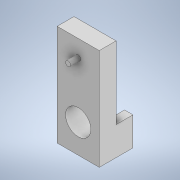
# Autodesk Inventor part: bottom_part
Saved by Autodesk Inventor 2021 (Build 250183000, 183)
## iProperties
Created: 2021-04-02
Part Number: bottom_part
Material: Generic
Document SubType Name: Modeling
Designer: Jawal
Density: 1 g/cm^3
Appearance: Default
Author: Jawal
Autodesk Inventor part; units mm, degrees
note: some values were not read from the file. Chosen so that the rebuilt part matches the saved one: direction of "Emboss1".
ref_plane "YZ Plane" through (0, 0, 0) normal (1, 0, 0) x (0, 1, 0)
ref_plane "XZ Plane" through (0, 0, 0) normal (0, 1, 0) x (-1, 0, 0)
ref_plane "XY Plane" through (0, 0, 0) normal (0, 0, 1) x (1, 0, 0)
sketch "Sketch1" plane through (0, 0, 0) normal (0, 0, 1) x (1, 0, 0)
  line L0 (-12.5, -12.5) -> (12.5, -12.5)
  line L1 (12.5, -12.5) -> (12.5, 47.5)
  line L2 (12.5, 47.5) -> (-12.5, 47.5)
  line L3 (-12.5, 47.5) -> (-12.5, -12.5)
  point P0 (0, 0)
  dimension "d0" = 60
  dimension "d1" = 25
  dimension "d2" = 12.5
  dimension "d5" = 12.5
  constraints: 8 end point, 2 parallel, 1 horizontal, 1 perpendicular
  measures "d0" distance of L0.end L1.end
  measures "d1" distance of L0.start L0.end
  measures "d2" distance from line of L3 point (0, 0)
  measures "d5" distance from line of L0 point (0, 0)
extrude "Extrusion1" add sketch "Sketch1" against normal blind 10
sketch "Sketch2" plane through (0, 0, 0) normal (0, 0, 1) x (1, 0, 0)
  circle A0 centre (0, 37.5) radius 1.5
  point P0 (0, 0)
  dimension "d8" = 3
  dimension "d29" = 37.5
  constraints: 1 centre point
  measures "d8" diameter of A0
  measures "d29" distance of point (0, 0) A0.centre
extrude "Extrusion2" add sketch "Sketch2" along normal blind 6
thread "Thread1" size "M3x0.5" class "6g" standard "ANSI Metric M Profile" full length
sketch "Sketch3" plane through (0, 0, -10) normal (0, 0, -1) x (-1, 0, 0)
  line L0 (-7.5, 4.5) -> (-12.5, 4.5)
  line L1 (-12.5, 47.5) -> (-12.5, -12.5) projected
  line L2 (-12.5, -12.5) -> (12.5, -12.5) projected
  line L3 (-12.5, -12.5) -> (12.5, -12.5)
  line L4 (12.5, -12.5) -> (12.5, 4.5)
  line L5 (12.5, -12.5) -> (12.5, 47.5) projected
  line L6 (7.5, 4.5) -> (12.5, 4.5)
  arc A0 (-7.5, 4.5) -> (7.5, 4.5) centre (0, 4.5) ccw
  point P0 (0, 0)
  dimension "d20" = 17
  dimension "d21" = 5
  dimension "d22" = 5
  dimension "d25" = 7.5
  constraints: 8 end point, 4 point on line, 2 horizontal, 2 point on circle, 1 centre point, 1 perpendicular
  measures "d20" distance of L2.end L4.end
  measures "d21" distance of L6.start L4.end
  measures "d22" distance of L0.start L0.end
  measures "d25" radius of A0
extrude "Extrusion3" add sketch "Sketch3" along normal blind 10
sketch "Sketch5" plane through (0, 0, 0) normal (0, 0, 1) x (1, 0, 0)
  circle A0 centre (0, 4.5) radius 7.5
  point P0 (0, 0)
  dimension "d26" = 15
  constraints: 1 centre point
  measures "d26" diameter of A0
extrude "Extrusion5" cut sketch "Sketch5" against normal blind 10
sketch "Sketch6" plane through (-12.5, -12.5, 0) normal (-1, 0, 0) x (0, 0, 1)
  line L0 (-17.643, 6.905) -> (1.6858, 6.905) construction
  line L1 (1.6858, 6.905) -> (1.6858, -1.4052) construction
  line L2 (1.6858, -1.4052) -> (-17.643, -1.4052) construction
  line L3 (-17.643, -1.4052) -> (-17.643, 6.905) construction
  line L4 (-17.3898, 4.3888) -> (-17.3898, 6.8888)
  line L5 (-17.3898, 6.8888) -> (-15.8257, 6.8888)
  line L6 (-15.8257, 6.8888) -> (-15.8257, 6.593)
  line L7 (-15.8257, 6.593) -> (-17.0575, 6.593)
  line L8 (-17.0575, 6.593) -> (-17.0575, 5.9082)
  line L9 (-17.0575, 5.9082) -> (-15.9088, 5.9082)
  line L10 (-15.9088, 5.9082) -> (-15.9088, 5.6124)
  line L11 (-15.9088, 5.6124) -> (-17.0575, 5.6124)
  line L12 (-17.0575, 5.6124) -> (-17.0575, 4.6846)
  line L13 (-17.0575, 4.6846) -> (-15.8257, 4.6846)
  line L14 (-15.8257, 4.6846) -> (-15.8257, 4.3888)
  line L15 (-15.8257, 4.3888) -> (-17.3898, 4.3888)
  line L16 (-14.0287, 4.3888) -> (-14.4157, 4.3888)
  line L17 (-14.4157, 4.3888) -> (-14.8715, 5.0938)
  line L18 (-14.8715, 5.0938) -> (-15.3395, 4.3888)
  line L19 (-15.3395, 4.3888) -> (-15.6981, 4.3888)
  line L20 (-15.6981, 4.3888) -> (-15.0478, 5.3187)
  line L21 (-15.0478, 5.3187) -> (-15.692, 6.2648)
  line L22 (-15.692, 6.2648) -> (-15.3051, 6.2648)
  line L23 (-15.3051, 6.2648) -> (-14.8513, 5.5658)
  line L24 (-14.8513, 5.5658) -> (-14.3873, 6.2648)
  line L25 (-14.3873, 6.2648) -> (-14.0287, 6.2648)
  line L26 (-14.0287, 6.2648) -> (-14.675, 5.3389)
  line L27 (-14.675, 5.3389) -> (-14.0287, 4.3888)
  line L28 (-13.4615, 4.3888) -> (-13.7775, 4.3888)
  line L29 (-13.7775, 4.3888) -> (-13.7775, 6.2648)
  line L30 (-13.7775, 6.2648) -> (-13.4615, 6.2648)
  line L31 (-13.4615, 6.2648) -> (-13.4615, 4.3888)
  line L32 (-13.4392, 6.5768) -> (-13.7978, 6.5768)
  line L33 (-13.7978, 6.5768) -> (-13.7978, 6.905)
  line L34 (-13.7978, 6.905) -> (-13.4392, 6.905)
  line L35 (-13.4392, 6.905) -> (-13.4392, 6.5768)
  spline S0 degree 2 poles (-12.4303, 4.3523) (-12.6876, 4.3523) (-12.9773, 4.6461) (-12.9773, 4.9641) knots 0 0 0 1 2 2 2
  line L36 (-12.9773, 4.9641) -> (-12.9773, 6.0034)
  line L37 (-12.9773, 6.0034) -> (-13.19, 6.0034)
  line L38 (-13.19, 6.0034) -> (-13.19, 6.2648)
  line L39 (-13.19, 6.2648) -> (-12.9773, 6.2648)
  line L40 (-12.9773, 6.2648) -> (-12.9773, 6.8037)
  line L41 (-12.9773, 6.8037) -> (-12.6612, 6.8037)
  line L42 (-12.6612, 6.8037) -> (-12.6612, 6.2648)
  line L43 (-12.6612, 6.2648) -> (-12.0798, 6.2648)
  line L44 (-12.0798, 6.2648) -> (-12.0798, 6.0034)
  line L45 (-12.0798, 6.0034) -> (-12.6612, 6.0034)
  line L46 (-12.6612, 6.0034) -> (-12.6612, 5.11)
  spline S1 degree 2 poles (-12.6612, 5.11) (-12.6612, 4.9682) (-12.6511, 4.8122) (-12.6167, 4.7453) knots 0 0 0 1 2 2 2
  spline S2 degree 2 poles (-12.6167, 4.7453) (-12.5883, 4.6866) (-12.4607, 4.6278) (-12.3513, 4.6278) knots 0 0 0 1 2 2 2
  spline S3 degree 2 poles (-12.3513, 4.6278) (-12.2743, 4.6278) (-12.1304, 4.6744) (-12.098, 4.6886) knots 0 0 0 1 2 2 2
  line L47 (-12.098, 4.6886) -> (-12.0798, 4.6886)
  line L48 (-12.0798, 4.6886) -> (-12.0798, 4.405)
  spline S4 degree 2 poles (-12.0798, 4.405) (-12.1689, 4.3807) (-12.3513, 4.3523) (-12.4303, 4.3523) knots 0 0 0 1 2 2 2
  line L49 (-8.814, 4.3888) -> (-9.2455, 4.3888)
  line L50 (-9.2455, 4.3888) -> (-10.0356, 5.3835)
  line L51 (-10.0356, 5.3835) -> (-10.4165, 5.3835)
  line L52 (-10.4165, 5.3835) -> (-10.4165, 4.3888)
  line L53 (-10.4165, 4.3888) -> (-10.7487, 4.3888)
  line L54 (-10.7487, 4.3888) -> (-10.7487, 6.8888)
  line L55 (-10.7487, 6.8888) -> (-10.1045, 6.8888)
  spline S5 degree 2 poles (-10.1045, 6.8888) (-9.8898, 6.8888) (-9.6, 6.8422) (-9.4684, 6.7571) knots 0 0 0 1 2 2 2
  spline S6 degree 2 poles (-9.4684, 6.7571) (-9.3367, 6.672) (-9.1847, 6.4066) (-9.1847, 6.2101) knots 0 0 0 1 2 2 2
  spline S7 degree 2 poles (-9.1847, 6.2101) (-9.1847, 5.9366) (-9.4643, 5.5658) (-9.7034, 5.4767) knots 0 0 0 1 2 2 2
  line L56 (-9.7034, 5.4767) -> (-8.814, 4.3888)
  spline S8 degree 2 poles (-9.5312, 6.1838) (-9.5312, 6.2932) (-9.6081, 6.4613) (-9.6892, 6.516) knots 0 0 0 1 2 2 2
  spline S9 degree 2 poles (-9.6892, 6.516) (-9.7601, 6.5626) (-9.9485, 6.6011) (-10.0863, 6.6011) knots 0 0 0 1 2 2 2
  line L57 (-10.0863, 6.6011) -> (-10.4165, 6.6011)
  line L58 (-10.4165, 6.6011) -> (-10.4165, 5.6611)
  line L59 (-10.4165, 5.6611) -> (-10.1248, 5.6611)
  spline S10 degree 2 poles (-10.1248, 5.6611) (-9.9809, 5.6611) (-9.752, 5.7117) (-9.673, 5.7907) knots 0 0 0 1 2 2 2
  spline S11 degree 2 poles (-9.673, 5.7907) (-9.6, 5.8596) (-9.5312, 6.0541) (-9.5312, 6.1838) knots 0 0 0 1 2 2 2
  spline S12 degree 2 poles (-7.5944, 4.5873) (-7.6329, 4.559) (-7.7625, 4.4577) (-7.8233, 4.4273) knots 0 0 0 1 2 2 2
  spline S13 degree 2 poles (-7.8233, 4.4273) (-7.9064, 4.3827) (-8.0624, 4.3361) (-8.2042, 4.3361) knots 0 0 0 1 2 2 2
  spline S14 degree 2 poles (-8.2042, 4.3361) (-8.3197, 4.3361) (-8.5283, 4.4232) (-8.6073, 4.5022) knots 0 0 0 1 2 2 2
  spline S15 degree 2 poles (-8.6073, 4.5022) (-8.6823, 4.5792) (-8.7735, 4.8061) (-8.7735, 4.9317) knots 0 0 0 1 2 2 2
  spline S16 degree 2 poles (-8.7735, 4.9317) (-8.7735, 5.1262) (-8.6094, 5.4017) (-8.4311, 5.4808) knots 0 0 0 1 2 2 2
  spline S17 degree 2 poles (-8.4311, 5.4808) (-8.2731, 5.5537) (-7.8436, 5.6084) (-7.5944, 5.6226) knots 0 0 0 1 2 2 2
  line L60 (-7.5944, 5.6226) -> (-7.5944, 5.6833)
  spline S18 degree 2 poles (-7.5944, 5.6833) (-7.5944, 5.7927) (-7.6612, 5.9285) (-7.722, 5.967) knots 0 0 0 1 2 2 2
  spline S19 degree 2 poles (-7.722, 5.967) (-7.7828, 6.0055) (-7.957, 6.0298) (-8.0502, 6.0298) knots 0 0 0 1 2 2 2
  spline S20 degree 2 poles (-8.0502, 6.0298) (-8.1596, 6.0298) (-8.4554, 5.965) (-8.6033, 5.9021) knots 0 0 0 1 2 2 2
  line L61 (-8.6033, 5.9021) -> (-8.6215, 5.9021)
  line L62 (-8.6215, 5.9021) -> (-8.6215, 6.2243)
  spline S21 degree 2 poles (-8.6215, 6.2243) (-8.5344, 6.2486) (-8.2082, 6.3094) (-8.0482, 6.3094) knots 0 0 0 1 2 2 2
  spline S22 degree 2 poles (-8.0482, 6.3094) (-7.8537, 6.3094) (-7.5883, 6.2486) (-7.4829, 6.1696) knots 0 0 0 1 2 2 2
  spline S23 degree 2 poles (-7.4829, 6.1696) (-7.3796, 6.0926) (-7.2783, 5.8474) (-7.2783, 5.6712) knots 0 0 0 1 2 2 2
  line L63 (-7.2783, 5.6712) -> (-7.2783, 4.3888)
  line L64 (-7.2783, 4.3888) -> (-7.5944, 4.3888)
  line L65 (-7.5944, 4.3888) -> (-7.5944, 4.5873)
  line L66 (-7.5944, 4.8507) -> (-7.5944, 5.3714)
  spline S24 degree 2 poles (-7.5944, 5.3714) (-7.7078, 5.3612) (-8.0502, 5.3268) (-8.1576, 5.2944) knots 0 0 0 1 2 2 2
  spline S25 degree 2 poles (-8.1576, 5.2944) (-8.2832, 5.2559) (-8.4473, 5.0958) (-8.4473, 4.954) knots 0 0 0 1 2 2 2
  spline S26 degree 2 poles (-8.4473, 4.954) (-8.4473, 4.7919) (-8.265, 4.6278) (-8.0907, 4.6278) knots 0 0 0 1 2 2 2
  spline S27 degree 2 poles (-8.0907, 4.6278) (-7.9428, 4.6278) (-7.6997, 4.7555) (-7.5944, 4.8507) knots 0 0 0 1 2 2 2
  line L67 (-4.7074, 4.3888) -> (-4.7074, 5.4747)
  spline S28 degree 2 poles (-4.7074, 5.4747) (-4.7074, 5.6043) (-4.7277, 5.8252) (-4.7601, 5.8859) knots 0 0 0 1 2 2 2
  spline S29 degree 2 poles (-4.7601, 5.8859) (-4.7925, 5.9528) (-4.9161, 6.0176) (-5.0235, 6.0176) knots 0 0 0 1 2 2 2
  spline S30 degree 2 poles (-5.0235, 6.0176) (-5.1207, 6.0176) (-5.3436, 5.8981) (-5.4611, 5.7846) knots 0 0 0 1 2 2 2
  spline S31 degree 2 poles (-5.4611, 5.7846) (-5.459, 5.7563) (-5.455, 5.6773) (-5.455, 5.6246) knots 0 0 0 1 2 2 2
  line L68 (-5.455, 5.6246) -> (-5.455, 4.3888)
  line L69 (-5.455, 4.3888) -> (-5.771, 4.3888)
  line L70 (-5.771, 4.3888) -> (-5.771, 5.4747)
  spline S32 degree 2 poles (-5.771, 5.4747) (-5.771, 5.6043) (-5.7913, 5.8252) (-5.8237, 5.8859) knots 0 0 0 1 2 2 2
  spline S33 degree 2 poles (-5.8237, 5.8859) (-5.8561, 5.9528) (-5.9797, 6.0176) (-6.0871, 6.0176) knots 0 0 0 1 2 2 2
  spline S34 degree 2 poles (-6.0871, 6.0176) (-6.1884, 6.0176) (-6.4133, 5.89) (-6.5186, 5.7907) knots 0 0 0 1 2 2 2
  line L71 (-6.5186, 5.7907) -> (-6.5186, 4.3888)
  line L72 (-6.5186, 4.3888) -> (-6.8346, 4.3888)
  line L73 (-6.8346, 4.3888) -> (-6.8346, 6.2648)
  line L74 (-6.8346, 6.2648) -> (-6.5186, 6.2648)
  line L75 (-6.5186, 6.2648) -> (-6.5186, 6.0581)
  spline S35 degree 2 poles (-6.5186, 6.0581) (-6.395, 6.1817) (-6.1519, 6.3175) (-6.006, 6.3175) knots 0 0 0 1 2 2 2
  spline S36 degree 2 poles (-6.006, 6.3175) (-5.8399, 6.3175) (-5.5826, 6.1655) (-5.5158, 5.9933) knots 0 0 0 1 2 2 2
  spline S37 degree 2 poles (-5.5158, 5.9933) (-5.3719, 6.1534) (-5.1004, 6.3175) (-4.9424, 6.3175) knots 0 0 0 1 2 2 2
  spline S38 degree 2 poles (-4.9424, 6.3175) (-4.8209, 6.3175) (-4.6223, 6.2425) (-4.5494, 6.1574) knots 0 0 0 1 2 2 2
  spline S39 degree 2 poles (-4.5494, 6.1574) (-4.4744, 6.0723) (-4.3914, 5.8171) (-4.3914, 5.6246) knots 0 0 0 1 2 2 2
  line L76 (-4.3914, 5.6246) -> (-4.3914, 4.3888)
  line L77 (-4.3914, 4.3888) -> (-4.7074, 4.3888)
  spline S40 degree 2 poles (-2.3756, 5.3774) (-2.3756, 4.9074) (-2.8233, 4.3523) (-3.1657, 4.3523) knots 0 0 0 1 2 2 2
  spline S41 degree 2 poles (-3.1657, 4.3523) (-3.3055, 4.3523) (-3.5202, 4.4171) (-3.6316, 4.484) knots 0 0 0 1 2 2 2
  line L78 (-3.6316, 4.484) -> (-3.6316, 3.6979)
  line L79 (-3.6316, 3.6979) -> (-3.9477, 3.6979)
  line L80 (-3.9477, 3.6979) -> (-3.9477, 6.2648)
  line L81 (-3.9477, 6.2648) -> (-3.6316, 6.2648)
  line L82 (-3.6316, 6.2648) -> (-3.6316, 6.0683)
  spline S42 degree 2 poles (-3.6316, 6.0683) (-3.5141, 6.1756) (-3.2265, 6.3175) (-3.0583, 6.3175) knots 0 0 0 1 2 2 2
  spline S43 degree 2 poles (-3.0583, 6.3175) (-2.7362, 6.3175) (-2.3756, 5.8069) (-2.3756, 5.3774) knots 0 0 0 1 2 2 2
  spline S44 degree 2 poles (-2.7017, 5.341) (-2.7017, 5.6631) (-2.9064, 6.0176) (-3.1353, 6.0176) knots 0 0 0 1 2 2 2
  spline S45 degree 2 poles (-3.1353, 6.0176) (-3.269, 6.0176) (-3.5202, 5.8981) (-3.6316, 5.8049) knots 0 0 0 1 2 2 2
  line L83 (-3.6316, 5.8049) -> (-3.6316, 4.7393)
  spline S46 degree 2 poles (-3.6316, 4.7393) (-3.5081, 4.6805) (-3.3318, 4.6359) (-3.2184, 4.6359) knots 0 0 0 1 2 2 2
  spline S47 degree 2 poles (-3.2184, 4.6359) (-2.9732, 4.6359) (-2.7017, 4.9966) (-2.7017, 5.341) knots 0 0 0 1 2 2 2
  point P0 (0, 12.5)
  constraints: 2 other
emboss "Emboss1" sketch "Sketch6" operation cut depth 1 direction (1, 0, 0)
equation "\"d2\" = 0.5 * d1"
body "Solid1"
